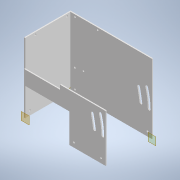
# Autodesk Inventor part: ShootingMech_Housing6
Saved by Autodesk Inventor 2020 (Build 240168000, 168)
## iProperties
Created: 2022-01-27
Part Number: ShootingMech_Housing6
Material: Generic
Document SubType Name: Modeling
Designer: danie
Density: 1 g/cm^3
Appearance: Default
Author: danie
Autodesk Inventor part; units mm, degrees
ref_plane "YZ Plane" through (0, 0, 0) normal (1, 0, 0) x (0, 1, 0)
ref_plane "XZ Plane" through (0, 0, 0) normal (0, 1, 0) x (-1, 0, 0)
ref_plane "XY Plane" through (0, 0, 0) normal (0, 0, 1) x (1, 0, 0)
ref_plane "Work Plane1" through (228.6, 0, -127) normal (0, 0, -1) x (-1, 0, 0)
sketch "Sketch5" plane through (228.6, 0, -127) normal (0, 0, -1) x (-1, 0, 0)
  line L0 (0, 0) -> (228.6, 0)
  line L1 (228.6, 0) -> (228.6, 194.818)
  line L2 (228.6, 194.818) -> (0, 194.818)
  line L3 (0, 194.818) -> (0, 0)
  circle A0 centre (549.0601, -0.0332) radius 2.1647 construction
  circle A1 centre (192.2498, 69.0594) radius 2.1647 construction
  arc A2 (37.5756, 109.1194) -> (31.2075, 73.1741) centre (549.0601, -0.0332) ccw construction
  arc A3 (33.8495, 109.9145) -> (27.435, 73.7074) centre (549.0601, -0.0332) ccw
  arc A4 (41.3017, 108.3242) -> (34.98, 72.6408) centre (549.0601, -0.0332) ccw
  arc A5 (41.3017, 108.3242) -> (33.8495, 109.9145) centre (37.5756, 109.1194) ccw
  arc A6 (27.435, 73.7074) -> (34.98, 72.6408) centre (31.2075, 73.1741) ccw
  line L4 (549.0601, -0.0332) -> (37.5756, 109.1194) construction
  line L5 (549.0601, -0.0332) -> (31.2075, 73.1741) construction
  arc A7 (14.9709, 119.3205) -> (7.984, 69.4017) centre (192.2498, 69.0594) ccw construction
  arc A8 (11.3053, 120.3597) -> (4.174, 69.4087) centre (192.2498, 69.0594) ccw
  arc A9 (18.6364, 118.2812) -> (11.794, 69.3946) centre (192.2498, 69.0594) ccw
  arc A10 (18.6364, 118.2812) -> (11.3053, 120.3597) centre (14.9709, 119.3205) ccw
  arc A11 (4.174, 69.4087) -> (11.794, 69.3946) centre (7.984, 69.4017) ccw
  circle A12 centre (192.2498, 69.0594) radius 2.1647
  circle A13 centre (216.5947, 65.3523) radius 2.2284
  line L6 (0, 0) -> (25.4, 0) construction
  line L7 (25.4, 0) -> (25.4, 25.4) construction
  line L8 (25.4, 25.4) -> (0, 25.4) construction
  line L9 (0, 25.4) -> (0, 0) construction
  line L10 (228.6, 0) -> (203.2, 0) construction
  line L11 (203.2, 0) -> (203.2, 25.4) construction
  line L12 (203.2, 25.4) -> (228.6, 25.4) construction
  line L13 (228.6, 25.4) -> (228.6, 0) construction
  line L14 (25.4, 25.4) -> (0, 0) construction
  line L15 (0, 25.4) -> (25.4, 0) construction
  line L16 (203.2, 25.4) -> (228.6, 0) construction
  line L17 (228.6, 25.4) -> (203.2, 0) construction
  circle A14 centre (12.7, 12.7) radius 2.3813
  circle A15 centre (215.9, 12.7) radius 2.3812
  line L18 (228.6, 194.818) -> (222.25, 194.818) construction
  line L19 (222.25, 194.818) -> (222.25, 169.418) construction
  line L20 (222.25, 169.418) -> (228.6, 169.418) construction
  line L21 (228.6, 169.418) -> (228.6, 194.818) construction
  line L22 (222.25, 194.818) -> (196.85, 194.818) construction
  line L23 (222.25, 169.418) -> (222.25, 194.818) construction
  line L24 (196.85, 194.818) -> (107.95, 194.818) construction
  line L25 (107.95, 194.818) -> (133.35, 194.818) construction
  line L26 (222.25, 194.818) -> (209.55, 194.818) construction
  line L27 (209.55, 194.818) -> (209.55, 182.118) construction
  line L28 (209.55, 182.118) -> (222.25, 182.118) construction
  line L29 (222.25, 182.118) -> (222.25, 194.818) construction
  line L30 (209.55, 194.818) -> (146.05, 194.818) construction
  line L31 (146.05, 194.818) -> (158.75, 194.818) construction
  line L32 (158.75, 194.818) -> (158.75, 182.118) construction
  line L33 (158.75, 182.118) -> (146.05, 182.118) construction
  line L34 (146.05, 182.118) -> (146.05, 194.818) construction
  line L35 (222.25, 194.818) -> (209.55, 182.118) construction
  line L36 (209.55, 194.818) -> (222.25, 182.118) construction
  line L37 (158.75, 194.818) -> (146.05, 182.118) construction
  line L38 (158.75, 182.118) -> (146.05, 194.818) construction
  circle A16 centre (215.9, 188.468) radius 2.3812
  circle A17 centre (152.4, 188.468) radius 2.3812
  dimension "d16" = 228.6
  dimension "d17" = 194.818
  dimension "d38" = 4
  dimension "d39" = 7.62
  dimension "d40" = 7.62
  dimension "d43" = 25.4
  dimension "d44" = 25.4
  dimension "d45" = 25.4
  dimension "d46" = 25.4
  dimension "d47" = 4.7625
  dimension "d48" = 4.7625
  dimension "d61" = 6.35
  dimension "d70" = 12.7
  dimension "d71" = 12.7
  dimension "d72" = 63.5
  dimension "d73" = 12.7
  dimension "d74" = 12.7
  dimension "d75" = 4.7625
  dimension "d76" = 4.7625
  constraints: 78 end point, 20 point on circle, 18 centre point, 12 parallel, 8 horizontal, 8 tangent, 6 perpendicular, 4 midpoint, 3 coincident, 2 point on line, 1 concentric
  measures "d16" distance of L2.end L1.end
  measures "d17" distance of L1.end L0.end
  measures "d38" angle of L4 L5
  measures "d39" diameter of A5
  measures "d40" diameter of A10
  measures "d43" distance of L8.end L7.end
  measures "d44" distance of L7.end L6.end
  measures "d45" distance of L11.end L12.end
  measures "d46" distance of L10.end L11.end
  measures "d47" diameter of A14
  measures "d48" diameter of A15
  measures "d61" distance of L20.end L19.end
  measures "d70" distance of L28.end L27.end
  measures "d71" distance of L27.end L26.end
  measures "d72" distance of L26.end L30.end
  measures "d73" distance of L32.end L33.end
  measures "d74" distance of L31.end L32.end
  measures "d75" diameter of A16
  measures "d76" diameter of A17
extrude "Extrusion5" add sketch "Sketch5" along normal blind 3.175
ref_plane "Work Plane2" through (0, 0.0003, -127) normal (-1, 0, 0) x (0, 0, 1)
sketch "Sketch6" plane through (0, 0.0003, -127) normal (-1, 0, 0) x (0, 0, 1)
  line L0 (-3.175, -0.0003) -> (-3.175, 194.8177) projected
  line L1 (-3.175, 194.8177) -> (127, 194.8177)
  line L2 (127, 194.8177) -> (127, -0.0003)
  line L3 (127, -0.0003) -> (-3.175, -0.0003)
  line L4 (-3.175, -0.0003) -> (-3.175, 194.8177)
  line L5 (0, -0.0003) -> (0, 194.8177) construction
  line L6 (0, -0.0003) -> (25.4, -0.0003) construction
  line L7 (25.4, -0.0003) -> (25.4, 25.3997) construction
  line L8 (25.4, 25.3997) -> (0, 25.3997) construction
  line L9 (0, 25.3997) -> (0, -0.0003) construction
  line L10 (127, -0.0003) -> (101.6, -0.0003) construction
  line L11 (101.6, -0.0003) -> (101.6, 25.3997) construction
  line L12 (101.6, 25.3997) -> (127, 25.3997) construction
  line L13 (127, 25.3997) -> (127, -0.0003) construction
  line L14 (0, -0.0003) -> (25.4, 25.3997) construction
  line L15 (0, 25.3997) -> (25.4, -0.0003) construction
  line L16 (101.6, -0.0003) -> (127, 25.3997) construction
  line L17 (101.6, 25.3997) -> (127, -0.0003) construction
  circle A0 centre (12.7, 12.6997) radius 2.3813
  circle A1 centre (114.3, 12.6997) radius 2.3813
  line L18 (0, 194.8177) -> (3.175, 194.8177) construction
  line L19 (3.175, 194.8177) -> (3.175, 169.4177) construction
  line L20 (3.175, 169.4177) -> (0, 169.4177) construction
  line L21 (0, 169.4177) -> (0, 194.8177) construction
  line L22 (3.175, 194.8177) -> (15.875, 194.8177) construction
  line L23 (15.875, 194.8177) -> (15.875, 182.1177) construction
  line L24 (15.875, 182.1177) -> (3.175, 182.1177) construction
  line L25 (3.175, 182.1177) -> (3.175, 194.8177) construction
  line L26 (15.875, 194.8177) -> (104.775, 194.8177) construction
  line L27 (104.775, 194.8177) -> (92.075, 194.8177) construction
  line L28 (92.075, 194.8177) -> (92.075, 182.1177) construction
  line L29 (92.075, 182.1177) -> (104.775, 182.1177) construction
  line L30 (104.775, 182.1177) -> (104.775, 194.8177) construction
  line L31 (3.175, 194.8177) -> (15.875, 182.1177) construction
  line L32 (3.175, 182.1177) -> (15.875, 194.8177) construction
  line L33 (92.075, 194.8177) -> (104.775, 182.1177) construction
  line L34 (104.775, 194.8177) -> (92.075, 182.1177) construction
  circle A2 centre (98.425, 188.4677) radius 2.3812
  circle A3 centre (9.525, 188.4677) radius 2.3813
  point P0 (-3.175, -0.0003)
  dimension "d49" = 25.4
  dimension "d50" = 25.4
  dimension "d51" = 25.4
  dimension "d52" = 25.4
  dimension "d53" = 4.7625
  dimension "d54" = 4.7625
  dimension "d77" = 3.175
  dimension "d78" = 25.4
  dimension "d79" = 12.7
  dimension "d80" = 12.7
  dimension "d81" = 88.9
  dimension "d82" = 12.7
  dimension "d83" = 12.7
  dimension "d84" = 4.7625
  dimension "d85" = 4.7625
  constraints: 66 end point, 12 parallel, 6 horizontal, 6 perpendicular, 4 centre point, 4 midpoint, 1 point on line
  measures "d49" distance of L8.end L7.end
  measures "d50" distance of L7.end L6.end
  measures "d51" distance of L11.end L12.end
  measures "d52" distance of L10.end L11.end
  measures "d53" diameter of A0
  measures "d54" diameter of A1
  measures "d77" distance of L19.end L20.end
  measures "d78" distance of L18.end L19.end
  measures "d79" distance of L23.end L24.end
  measures "d80" distance of L22.end L23.end
  measures "d81" distance of L22.end L26.end
  measures "d82" distance of L29.end L28.end
  measures "d83" distance of L28.end L27.end
  measures "d84" diameter of A2
  measures "d85" diameter of A3
extrude "Extrusion6" add sketch "Sketch6" along normal blind 3.175
ref_plane "Work Plane4" through (0, 0.0003, 0) normal (0, 0, 1) x (1, 0, 0)
sketch "Sketch7" plane through (0, 0.0003, 0) normal (0, 0, 1) x (1, 0, 0)
  line L0 (228.6, -0.0003) -> (228.6, 0) projected
  line L1 (228.6, -0.0003) -> (127, -0.0003)
  line L2 (127, -0.0003) -> (127, 194.8177)
  line L3 (127, 194.8177) -> (228.6, 194.8177)
  line L4 (228.6, 194.8177) -> (228.6, -0.0003)
  line L5 (228.6, -0.0003) -> (-3.175, -0.0003) projected
  line L6 (228.6, -0.0003) -> (127, -0.0003)
  line L7 (127, -0.0003) -> (127, 133.3497)
  line L8 (127, 133.3497) -> (228.6, 133.3497)
  line L9 (228.6, 133.3497) -> (228.6, -0.0003)
  arc A0 (217.2947, 120.3594) -> (209.9636, 118.281) centre (213.6291, 119.3202) ccw projected
  arc A1 (216.806, 69.3943) -> (209.9636, 118.281) centre (36.3502, 69.0591) ccw projected
  arc A2 (224.426, 69.4085) -> (217.2947, 120.3594) centre (36.3502, 69.0591) ccw projected
  arc A3 (216.806, 69.3943) -> (224.426, 69.4085) centre (220.616, 69.4014) ccw projected
  arc A4 (194.7505, 109.9143) -> (187.2983, 108.324) centre (191.0244, 109.1191) ccw projected
  arc A5 (193.62, 72.6406) -> (187.2983, 108.324) centre (-320.4601, -0.0334) ccw projected
  arc A6 (201.165, 73.7072) -> (194.7505, 109.9143) centre (-320.4601, -0.0334) ccw projected
  arc A7 (193.62, 72.6406) -> (201.165, 73.7072) centre (197.3925, 73.1739) ccw projected
  line L10 (127, -0.0003) -> (152.4, -0.0003) construction
  line L11 (152.4, -0.0003) -> (152.4, 25.3997) construction
  line L12 (152.4, 25.3997) -> (127, 25.3997) construction
  line L13 (127, 25.3997) -> (127, -0.0003) construction
  line L14 (228.6, 194.8177) -> (228.6, -0.0003) construction
  line L15 (228.6, -0.0003) -> (203.2, -0.0003) construction
  line L16 (203.2, -0.0003) -> (203.2, 25.3997) construction
  line L17 (203.2, 25.3997) -> (228.6, 25.3997) construction
  line L18 (228.6, 25.3997) -> (228.6, -0.0003) construction
  line L19 (127, 25.3997) -> (152.4, -0.0003) construction
  line L20 (152.4, 25.3997) -> (127, -0.0003) construction
  line L21 (228.6, -0.0003) -> (-3.175, -0.0003) construction
  line L22 (203.2, 25.3997) -> (228.6, -0.0003) construction
  line L23 (228.6, -0.0003) -> (228.6, 25.3997) construction
  line L24 (228.6, 25.3997) -> (203.2, -0.0003) construction
  circle A8 centre (139.7, 12.6997) radius 2.3813
  circle A9 centre (215.9, 12.6997) radius 2.3813
  line L25 (0, -0.0003) -> (0, 194.8177) projected
  line L26 (0, 121.2789) -> (127, 121.2789)
  line L27 (127, 121.2789) -> (127, 104.7109)
  line L28 (0, 104.7109) -> (0, 121.2789)
  line L29 (127, 133.3497) -> (100.9092, 133.3497)
  line L30 (100.9092, 133.3497) -> (100.9092, 121.2789)
  line L31 (100.9092, 121.2789) -> (127, 121.2789)
  line L32 (127, 121.2789) -> (127, 133.3497)
  line L33 (0, 121.2789) -> (127, 121.2789)
  line L34 (127, 121.2789) -> (127, 81.6877)
  line L35 (127, 81.6877) -> (0, 81.6877)
  line L36 (0, 81.6877) -> (0, 121.2789)
  line L37 (0, 121.2789) -> (-3.175, 121.2789)
  line L38 (-3.175, 121.2789) -> (-3.175, 81.6877)
  line L39 (-3.175, 81.6877) -> (0, 81.6877)
  line L40 (0, 81.6877) -> (0, 121.2789)
  point P0 (127, 133.3497)
  dimension "d22" = 101.6
  dimension "d23" = 194.818
  dimension "d26" = 101.6
  dimension "d27" = 133.35
  dimension "d55" = 25.4
  dimension "d56" = 25.4
  dimension "d57" = 25.4
  dimension "d58" = 25.4
  dimension "d59" = 4.7625
  dimension "d60" = 4.7625
  constraints: 72 end point, 15 parallel, 8 horizontal, 8 perpendicular, 4 point on line, 2 centre point, 2 midpoint
  measures "d22" distance of L2.end L3.end
  measures "d23" distance of L1.end L2.end
  measures "d26" distance of L7.end L8.end
  measures "d27" distance of L6.end L7.end
  measures "d55" distance of L12.end L11.end
  measures "d56" distance of L11.end L10.end
  measures "d57" distance of L16.end L17.end
  measures "d58" distance of L15.end L16.end
  measures "d59" diameter of A8
  measures "d60" diameter of A9
extrude "Extrusion7" add sketch "Sketch7" along normal blind 3.175 contours L1 L2 L8 L4 | L35 L25 L26 L2 | L2 L26 L30 L29 | L39 L38 L37 L25
ref_plane "Work Plane3" through (0, 0.0003, 0) normal (0, 0, 1) x (1, 0, 0)
sketch "Sketch8" plane through (0, 0.0003, 0) normal (0, 0, 1) x (1, 0, 0)
  line L0 (18.6832, 91.7066) -> (0, 110.3898)
  line L1 (0, 0) -> (0, 194.8177) projected
  line L2 (18.6832, 91.7066) -> (45.1053, 91.7066) construction
  line L3 (0, 110.3898) -> (0, 113.5648) construction
  line L4 (0, 113.5648) -> (21.8582, 91.7066)
  line L5 (0, 113.5648) -> (0, 110.3898) construction
  line L6 (18.6832, 91.7066) -> (21.8582, 91.7066) construction
  line L7 (18.6832, 91.7066) -> (21.8582, 91.7066)
  line L8 (0, 113.5648) -> (0, 110.3898)
  line L9 (18.6832, 91.7066) -> (16.4382, 93.9517)
  line L10 (18.6832, 91.7066) -> (21.8582, 91.7066) construction
  line L11 (18.6832, 91.7066) -> (0, 91.7066)
  line L12 (18.6832, 91.7066) -> (37.3664, 91.7066) construction
  line L13 (0, 91.7066) -> (0, 94.8816)
  line L14 (0, 94.8816) -> (15.5082, 94.8816)
  point P0 (0, -0.0003)
  dimension "d28" = 135
  dimension "d29" = 3.175
  dimension "d30" = 45
  dimension "d31" = 3.175
  dimension "d32" = 135
  dimension "d33" = 180
  dimension "d34" = 3.175
  dimension "d35" = 90
  constraints: 28 end point, 5 point on line, 3 collinear, 3 equal length, 3 horizontal, 2 perpendicular
  measures "d28" angle of L2 L0
  measures "d29" distance of L0.end L3.end
  measures "d30" angle of L3 L4
  measures "d31" distance of L0.start L9.end
  measures "d32" angle of L10 L9
  measures "d33" angle of L11 L12
  measures "d34" distance of L11.end L13.end
  measures "d35" angle of L11 L13
extrude "Extrusion8" [suppressed]
body "Solid1"
